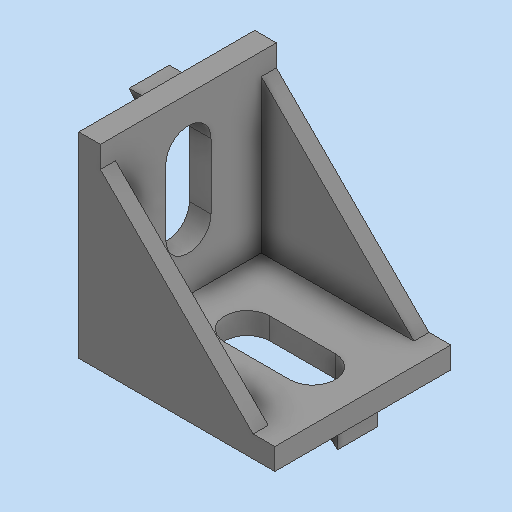
# Autodesk Inventor part: Bracket - Cast 90 deg corner 4040
Saved by Autodesk Inventor 2023.2 (Build 272271000, 271)
## iProperties
Created: 2023-11-22
Part Number: Bracket - Cast 90 deg corner 4040
Material: Generisch
Document SubType Name: Modeling
Designer: Nils Bade
Density: 1 g/cm^3
Appearance: Vorgabe
Author: Nils Bade
Autodesk Inventor part; units mm, degrees
ref_plane "YZ Plane" through (0, 0, 0) normal (1, 0, 0) x (0, 1, 0)
ref_plane "XY Plane" through (0, 0, 0) normal (0, 0, 1) x (1, 0, 0)
sketch "Skizze1" plane through (0, 0, 0) normal (0, 0, 1) x (1, 0, 0)
  line L0 (-12, 0) -> (47.5, 0) projected
  line L1 (0, 47.5) -> (0, -12) projected
  line L2 (39, 0) -> (39, 4.3)
  line L3 (39, 4.3) -> (34.6772, 4.3)
  line L4 (34.6772, 4.3) -> (4.3, 34.6772)
  line L5 (4.3, 34.6772) -> (4.3, 39)
  line L6 (4.3, 39) -> (0, 39)
  line L7 (0, 39) -> (0, 0)
  line L8 (0, 0) -> (39, 0)
  line L9 (34.6772, 4.3) -> (4.3, 4.3)
  line L10 (4.3, 4.3) -> (4.3, 34.6772)
  line L11 (0, 38) -> (-3.5, 38)
  line L12 (-3.5, 38) -> (0, 33.8289)
  line L13 (0, 4.1711) -> (-3.5, 0)
  line L14 (0, 0) -> (-3.5, 0)
  line L15 (0, 0) -> (0, -3.5)
  line L16 (0, -3.5) -> (4.1711, 0)
  line L17 (38, 0) -> (38, -3.5)
  line L18 (38, -3.5) -> (33.8289, 0)
  dimension "d0" = 39
  dimension "d1" = 39
  dimension "d2" = 4.3
  dimension "d3" = 4.3
  dimension "d4" = 45
  dimension "d7" = 40
  dimension "d8" = 40
  dimension "d9" = 40
  dimension "d10" = 40
  dimension "d11" = 3.5
  dimension "d12" = 3.5
  dimension "d13" = 3.5
  dimension "d14" = 3.5
  dimension "d15" = 1
  dimension "d16" = 1
  constraints: 34 end point, 10 point on line, 3 collinear, 3 perpendicular, 2 horizontal, 2 vertical, 1 parallel
  measures "d0" distance between parallel lines of L0 L6
  measures "d1" distance between parallel lines of L1 L2
  measures "d2" distance between parallel lines of L0 L3
  measures "d3" distance between parallel lines of L1 L5
  measures "d4" angle of L0 L4
  measures "d7" angle of L0 L18
  measures "d8" angle of L8 L16
  measures "d9" angle of L7 L13
  measures "d10" angle of L7 L12
  measures "d11" distance of L11.start L11.end
  measures "d12" distance of L7.end L13.end
  measures "d13" distance of L7.end L15.end
  measures "d14" distance of L17.start L17.end
  measures "d15" distance between parallel lines of L2 L17
  measures "d16" distance between parallel lines of L6 L11
extrude "Extrusion1" add sketch "Skizze1" along normal mid plane 35 contours L1 L6 L5 L10 L9 L3 L2 L0
extrude "Extrusion2" add sketch "Skizze1" along normal mid plane 8 contours L13 L1 L0 | L0 L16 L1 | L12 L11 L1 | L0 L17 L18
extrude "Extrusion3" add sketch "Skizze1" against normal blind 3 from surface at 17.5 contours L4 L9 L10
extrude "Extrusion4" add sketch "Skizze1" along normal blind 3 from surface at -17.5 contours L4 L9 L10
sketch "Skizze2" plane through (4.3, 39, 17.5) normal (1, 0, 0) x (0, 0, -1)
  line L0 (0, 0) -> (35, 0) projected
  line L1 (0, -4.3228) -> (0, 0) projected
  line L2 (0, -4.3228) -> (3, -4.3228) projected
  line L3 (3, -34.7) -> (3, -4.3228) projected
  line L4 (32, -34.7) -> (3, -34.7) projected
  line L5 (32, -4.3228) -> (32, -34.7) projected
  line L6 (32, -4.3228) -> (35, -4.3228) projected
  line L7 (35, 0) -> (35, -4.3228) projected
  line L8 (32, -4.3228) -> (35, -4.3228) construction
  line L9 (0, -4.3228) -> (3, -4.3228) construction
  line L10 (32, -34.7) -> (3, -34.7) construction
  line L11 (17.5, -23) -> (17.5, -10) construction
  line L12 (22, -23) -> (22, -10)
  line L13 (13, -10) -> (13, -23)
  arc A0 (13, -23) -> (22, -23) centre (17.5, -23) ccw
  arc A1 (22, -10) -> (13, -10) centre (17.5, -10) ccw
  line L14 (35, 0) -> (0, 0) construction
  line L15 (17.5, 0) -> (17.5, -49.0584) construction
  point P0 (17.5, -39)
  point P1 (17.5, -16.5)
  point P2 (17.5, -27.5)
  point P3 (17.5, -5.5)
  dimension "d23" = 6.5
  dimension "d24" = 9
  dimension "d25" = 22
  dimension "d26" = 5.5
  constraints: 10 end point, 6 point on circle, 4 tangent, 2 centre point, 2 midpoint, 2 vertical, 1 parallel, 1 point on line
  measures "d23" distance of point (17.5, -16.5) L11.end
  measures "d24" diameter of A1
  measures "d25" distance of point (17.5, -27.5) point (17.5, -5.5)
  measures "d26" distance from line of L14 point (17.5, -5.5)
extrude "Extrusion5" cut sketch "Skizze2" against normal blind 5 contours A0 L13 A1 L12
ref_plane "Arbeitsebene1" through (4.3, 4.3, 0) normal (-0.7071, 0.7071, 0) x (0, 0, 1)
mirror "Spiegeln1" about plane through (4.3, 4.3, 0) normal (-0.7071, 0.7071, 0) of "Extrusion5"
equation "\"d12\" = d11"
equation "\"d13\" = d11"
equation "\"d14\" = d11"
